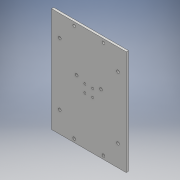
# Autodesk Inventor part: base superior
Saved by Autodesk Inventor 2018 (Build 220112000, 112)
## iProperties
Created: 2019-05-16
Part Number: base superior
Material: Generic
Document SubType Name: Modeling
Designer: JLVega003
Density: 1 g/cm^3
Appearance: Default
Author: JLVega003
Autodesk Inventor part; units mm, degrees
ref_plane "YZ Plane" through (0, 0, 0) normal (1, 0, 0) x (0, 1, 0)
ref_plane "XZ Plane" through (0, 0, 0) normal (0, 1, 0) x (-1, 0, 0)
ref_plane "XY Plane" through (0, 0, 0) normal (0, 0, 1) x (1, 0, 0)
sketch "Sketch1" plane through (0, 0, 0) normal (0, 1, 0) x (-1, 0, 0)
  line L0 (53.5, 75) -> (-53.5, 75)
  line L1 (-53.5, 75) -> (-53.5, -75)
  line L2 (-53.5, -75) -> (53.5, -75)
  line L3 (53.5, -75) -> (53.5, 75)
  line L4 (74.9, 0) -> (-74.9, 0) projected
  line L5 (0, -105) -> (0, 105) projected
  point P0 (0, 0)
  point P1 (0, 75)
  point P2 (53.5, 0)
  dimension "d0" = 150
  dimension "d1" = 107
  constraints: 8 end point, 2 midpoint, 2 parallel, 2 point on line, 1 horizontal, 1 perpendicular
  measures "d0" distance between parallel lines of L2 L0
  measures "d1" distance between parallel lines of L1 L3
extrude "Extrusion1" add sketch "Sketch1" along normal blind 3.175
sketch "Sketch2" plane through (0, 3.175, 0) normal (0, 1, 0) x (1, 0, 0)
  line L0 (-53.5, -75) -> (53.5, -75) projected
  line L1 (-53.5, 75) -> (-53.5, -75) projected
  line L2 (53.5, 75) -> (-53.5, 75) projected
  line L3 (0, 105) -> (0, -105) projected
  line L4 (-21, -70) -> (21, -70) construction
  line L5 (21, -70) -> (21, 70) construction
  line L6 (21, 70) -> (-21, 70) construction
  line L7 (-21, 70) -> (-21, -70) construction
  line L8 (-41.75, -44.5) -> (41.75, -44.5) construction
  line L9 (41.75, -44.5) -> (41.75, 44.5) construction
  line L10 (41.75, 44.5) -> (-41.75, 44.5) construction
  line L11 (-41.75, 44.5) -> (-41.75, -44.5) construction
  line L12 (-17.5, -10.5) -> (17.5, -10.5) construction
  line L13 (-74.9, 0) -> (74.9, 0) projected
  circle A0 centre (0, 0) radius 8 construction
  line L14 (5.6569, 5.6569) -> (-5.6569, -5.6569) construction
  line L15 (5.6569, -5.6569) -> (-5.6569, 5.6569) construction
  point P0 (0, -10.5)
  point P1 (0, -44.5)
  point P2 (-41.75, 0)
  point P3 (-21, 0)
  point P4 (0, -70)
  point P5 (-5.6569, -5.6569)
  point P6 (-5.6569, 5.6569)
  point P7 (5.6569, -5.6569)
  point P8 (5.6569, 5.6569)
  dimension "d31" = 64.5
  dimension "d34" = 35
  dimension "d35" = 30.5
  dimension "d36" = 11.75
  dimension "d37" = 5
  dimension "d38" = 42
  dimension "d54" = 16
  dimension "d55" = 45
  constraints: 22 end point, 14 coincident, 11 midpoint, 5 point on line, 4 parallel, 4 point on circle, 3 horizontal, 3 perpendicular, 1 centre point
  measures "d31" distance between parallel lines of L12 L0
  measures "d34" distance of L12.start L12.end
  measures "d35" distance between parallel lines of L8 L0
  measures "d36" distance between parallel lines of L11 L1
  measures "d37" distance between parallel lines of L4 L0
  measures "d38" distance between parallel lines of L5 L7
  measures "d54" diameter of A0
  measures "d55" angle of L13 L14
hole "Hole3" at (-41.75, 3.175, 44.5) at (-21, 3.175, 70) at (21, 3.175, 70) at (41.75, 3.175, 44.5) at (41.75, 3.175, -44.5) at (21, 3.175, -70) at (-21, 3.175, -70) at (-41.75, 3.175, -44.5) at (-17.5, 3.175, 10.5) at (17.5, 3.175, 10.5) direction (0, -1, 0) diameter 4 end through all
hole "Hole4" at (-5.6569, 3.175, 5.6569) at (-5.6569, 3.175, -5.6569) at (5.6569, 3.175, 5.6569) at (5.6569, 3.175, -5.6569) direction (0, -1, 0) diameter 3 end through all
body "Solid1"
